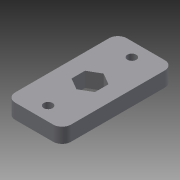
# Autodesk Inventor part: hex_plate
Saved by Autodesk Inventor 2015 (Build 190159000, 159)
## iProperties
Created: 2015-12-01
Part Number: hex_plate
Material: Generic
Document SubType Name: Modeling
Designer: jufranz
Density: 1 g/cm^3
Appearance: Default
Author: jufranz
Autodesk Inventor part; units mm, degrees
ref_plane "YZ Plane" through (0, 0, 0) normal (1, 0, 0) x (0, 1, 0)
ref_plane "XZ Plane" through (0, 0, 0) normal (0, 1, 0) x (-1, 0, 0)
ref_plane "XY Plane" through (0, 0, 0) normal (0, 0, 1) x (1, 0, 0)
sketch "Sketch1" plane through (0, 0, 0) normal (0, 1, 0) x (-1, 0, 0)
  line L0 (10, 20) -> (-10, 20)
  line L1 (-10, 20) -> (-10, -20)
  line L2 (-10, -20) -> (10, -20)
  line L3 (10, -20) -> (10, 20)
  point P0 (0, 0)
  point P1 (10, 0)
  point P2 (0, 20)
  dimension "d0" = 20
  dimension "d1" = 40
  constraints: 8 end point, 2 midpoint, 2 parallel, 1 horizontal, 1 horizontal alignment, 1 perpendicular, 1 vertical alignment
  measures "d0" distance of L0.start L0.end
  measures "d1" distance of L2.end L0.start
extrude "Extrusion1" add sketch "Sketch1" along normal blind 5.334
sketch "Sketch2" plane through (0, 5.334, 0) normal (0, 1, 0) x (1, 0, 0)
  line L0 (0, 4.8497) -> (4.2, 2.4249)
  line L1 (4.2, 2.4249) -> (4.2, -2.4249)
  line L2 (4.2, -2.4249) -> (0, -4.8497)
  line L3 (0, -4.8497) -> (-4.2, -2.4249)
  line L4 (-4.2, -2.4249) -> (-4.2, 2.4249)
  line L5 (-4.2, 2.4249) -> (0, 4.8497)
  point P0 (0, 0)
  point P1 (0, 0)
  dimension "d4" = 8.4
  constraints: 12 end point, 1 coincident, 13 other
  measures "d4" distance between parallel lines of L1 L4
extrude "Extrusion2" cut sketch "Sketch2" against normal through all
sketch "Sketch3" plane through (0, 5.334, 0) normal (0, 1, 0) x (1, 0, 0)
  point P0 (0, 0)
  point P1 (0, -15)
  point P2 (0, 15)
  dimension "d7" = 30
  dimension "d8" = 15
  constraints: 2 vertical alignment
  measures "d7" distance of point (0, 15) point (0, -15)
  measures "d8" distance of point (0, 0) point (0, 15)
hole "Hole1" at (0, 5.334, 15) at (0, 5.334, -15) direction (0, -1, 0) diameter 3.2 end through all
fillet "Fillet1" radius 3.175 4 edges at (-10, 2.667, 20) (10, 2.667, 20) (10, 2.667, -20) (-10, 2.667, -20)
equation "\"d8\" = 0.5 * d7"
body "Solid1"
